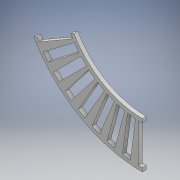
# Autodesk Inventor part: stator-60deg-holder
Saved by Autodesk Inventor 2018 (Build 220112000, 112)
## iProperties
Created: 2024-05-02
Part Number: stator-60deg-holder
Material: Generic
Document SubType Name: Modeling
Designer: neo
Density: 1 g/cm^3
Appearance: Default
Author: neo
Autodesk Inventor part; units mm, degrees
ref_plane "YZ Plane" through (0, 0, 0) normal (1, 0, 0) x (0, 1, 0)
ref_plane "XZ Plane" through (0, 0, 0) normal (0, 1, 0) x (-1, 0, 0)
ref_plane "XY Plane" through (0, 0, 0) normal (0, 0, 1) x (1, 0, 0)
sketch "Sketch1" plane through (0, 0, 0) normal (0, 1, 0) x (-1, 0, 0)
  circle A0 centre (0, 0) radius 102.5 construction
  circle A1 centre (0, 0) radius 162.5 construction
  line L0 (0, -102.5) -> (0, -162.5)
  line L1 (0, 0) -> (140.7291, -81.25)
  arc A2 (0, -102.5) -> (88.7676, -51.25) centre (0, 0) ccw
  arc A3 (0, -162.5) -> (140.7291, -81.25) centre (0, 0) ccw
  dimension "d1" = 205
  dimension "d2" = 60
  dimension "d0" = 60
  constraints: 4 coincident, 4 end point, 4 point on circle, 2 centre point, 2 vertical alignment, 1 point on line, 1 vertical, 4 other
  measures "d0" angle of L0 L1
extrude "Extrusion1" add sketch "Sketch1" along normal blind 5
sketch "Sketch2" plane through (0, 5, 0) normal (0, 1, 0) x (1, 0, 0)
  line L0 (0, 102.5) -> (0, 162.5) projected
  arc A0 (0, 162.5) -> (-140.7291, 81.25) centre (0, 0) ccw projected
  line L1 (-140.7291, 81.25) -> (-88.7676, 51.25) projected
  arc A1 (0, 102.5) -> (-88.7676, 51.25) centre (0, 0) ccw projected
  line L2 (0, 102.5) -> (0, 162.5) projected
  line L3 (0, 102.5) -> (-33.162, 102.5)
  arc A2 (0, 102.5) -> (-88.7676, 51.25) centre (0, 0) ccw projected
  line L4 (0, 162.5) -> (-30.7981, 162.5)
  arc A3 (0, 162.5) -> (-140.7291, 81.25) centre (0, 0) ccw projected
  line L5 (-16.4331, 132.5) -> (15.7518, 132.5)
  line L6 (-5.2, 107.5) -> (5.2, 107.5)
  line L7 (5.2, 107.5) -> (5.2, 157.5)
  line L8 (5.2, 157.5) -> (-5.2, 157.5)
  line L9 (-5.2, 157.5) -> (-5.2, 107.5)
  line L10 (-15.4024, 156.8313) -> (-25.7134, 155.4738)
  line L11 (-19.1871, 105.9016) -> (-8.8761, 107.2591)
  line L12 (-8.8761, 107.2591) -> (-15.4024, 156.8313)
  line L13 (-25.7134, 155.4738) -> (-19.1871, 105.9016)
  line L14 (-35.7412, 153.4792) -> (-45.7868, 150.7875)
  line L15 (-32.8459, 102.4912) -> (-22.8002, 105.1829)
  line L16 (-22.8002, 105.1829) -> (-35.7412, 153.4792)
  line L17 (-45.7868, 150.7875) -> (-32.8459, 102.4912)
  line L18 (-55.4685, 147.501) -> (-65.0768, 143.5211)
  line L19 (-45.9426, 97.3271) -> (-36.3343, 101.307)
  line L20 (-36.3343, 101.307) -> (-55.4685, 147.501)
  line L21 (-65.0768, 143.5211) -> (-45.9426, 97.3271)
  line L22 (-74.2467, 138.999) -> (-83.2533, 133.799)
  line L23 (-58.2533, 90.4977) -> (-49.2467, 95.6977)
  line L24 (-49.2467, 95.6977) -> (-74.2467, 138.999)
  line L25 (-83.2533, 133.799) -> (-58.2533, 90.4977)
  line L26 (-91.7545, 128.1187) -> (-100.0054, 121.7876)
  line L27 (-69.5673, 82.1199) -> (-61.3164, 88.451)
  line L28 (-61.3164, 88.451) -> (-91.7545, 128.1187)
  line L29 (-100.0054, 121.7876) -> (-69.5673, 82.1199)
  line L30 (-107.6924, 115.0463) -> (-115.0463, 107.6924)
  line L31 (-79.6909, 72.337) -> (-72.337, 79.6909)
  line L32 (-72.337, 79.6909) -> (-107.6924, 115.0463)
  line L33 (-115.0463, 107.6924) -> (-79.6909, 72.337)
  line L34 (-121.7876, 100.0054) -> (-128.1187, 91.7545)
  line L35 (-88.451, 61.3164) -> (-82.1199, 69.5673)
  line L36 (-82.1199, 69.5673) -> (-121.7876, 100.0054)
  line L37 (-128.1187, 91.7545) -> (-88.451, 61.3164)
  line L38 (-133.799, 83.2533) -> (-138.999, 74.2467)
  line L39 (-95.6977, 49.2467) -> (-90.4977, 58.2533)
  line L40 (-90.4977, 58.2533) -> (-133.799, 83.2533)
  line L41 (-138.999, 74.2467) -> (-95.6977, 49.2467)
  dimension "d8" = 10.4
  dimension "d9" = 50
  dimension "d12" = 60
  constraints: 78 end point, 4 horizontal, 3 tangent, 2 parallel, 1 perpendicular, 68 other
  measures "d8" distance of L7.end L8.end
  measures "d9" distance of L8.end L6.start
extrude "Extrusion2" cut sketch "Sketch2" against normal through all contours L6 L9 L5 L0 | L0 L5 L7 L6 | L5 L9 L8 L0 | L0 L8 L7 L5 | L39 L41 L38 L1 | L1 L38 L40 L39 | L15 L17 L3 | L3 L17 L14 L16 L15 | L12 L11 L13 L10 | L20 L19 L21 L18 | L24 L23 L25 L22 | L28 L27 L29 L26 | L32 L31 L33 L30 | L36 L35 L37 L34
body "Solid1"
